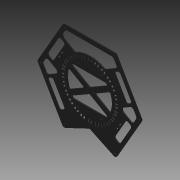
# Autodesk Inventor part: Bottom Plate
Saved by Autodesk Inventor 2015 (Build 190159000, 159)
## iProperties
Created: 2016-10-01
Part Number: Bottom Plate
Material: PVC, Unplasticized
Document SubType Name: Modeling
Designer: James Yelland
Density: 1.29 g/cm^3
Appearance: Smooth - White
Mass: 43.6601 g
Surface Area: 401.333 cm^2
Volume: 33.8451 cm^3
Author: James Yelland
Autodesk Inventor part; units mm, degrees
ref_plane "YZ Plane" through (0, 0, 0) normal (1, 0, 0) x (0, 1, 0)
ref_plane "XZ Plane" through (0, 0, 0) normal (0, 1, 0) x (-1, 0, 0)
ref_plane "XY Plane" through (0, 0, 0) normal (0, 0, 1) x (1, 0, 0)
sketch "Sketch1" plane through (0, 0, 0) normal (0, 1, 0) x (-1, 0, 0)
  line L0 (72.6878, -41.9663) -> (62.1878, -60.1529)
  line L1 (72.6878, -41.9663) -> (83.1878, -23.7798)
  line L2 (81.7237, -18.3157) -> (77.3936, -15.8157)
  line L3 (71.9295, -17.2797) -> (50.9295, -53.6529)
  line L4 (52.3936, -59.117) -> (56.7237, -61.617)
  arc A0 (56.7237, -61.617) -> (62.1878, -60.1529) centre (58.7237, -58.1529) ccw
  arc A1 (50.9295, -53.6529) -> (52.3936, -59.117) centre (54.3936, -55.6529) ccw
  arc A2 (77.3936, -15.8157) -> (71.9295, -17.2797) centre (75.3936, -19.2798) ccw
  arc A3 (83.1878, -23.7798) -> (81.7237, -18.3157) centre (79.7237, -21.7798) ccw
  line L5 (55.5994, -35.5644) -> (57.3314, -36.5644)
  line L6 (57.3314, -36.5644) -> (54.8314, -40.8945)
  line L7 (53.0994, -39.8945) -> (55.5994, -35.5644)
  line L8 (54.8314, -40.8945) -> (53.0994, -39.8945)
  line L9 (61.0994, -26.0381) -> (58.5994, -30.3683)
  line L10 (60.3314, -31.3683) -> (62.8314, -27.0381)
  line L11 (58.5994, -30.3683) -> (60.3314, -31.3683)
  line L12 (62.8314, -27.0381) -> (61.0994, -26.0381)
  line L13 (-72.6878, -41.9663) -> (-83.1878, -23.7798)
  line L14 (-72.6878, -41.9663) -> (-62.1878, -60.1529)
  line L15 (-56.7237, -61.617) -> (-52.3936, -59.117)
  line L16 (-50.9295, -53.6529) -> (-71.9294, -17.28)
  line L17 (-77.3936, -15.8157) -> (-81.7237, -18.3157)
  arc A4 (-81.7237, -18.3157) -> (-83.1878, -23.7798) centre (-79.7237, -21.7798) ccw
  arc A5 (-71.9294, -17.28) -> (-77.3936, -15.8157) centre (-75.3936, -19.2798) ccw
  arc A6 (-52.3936, -59.117) -> (-50.9295, -53.6529) centre (-54.3936, -55.6529) ccw
  arc A7 (-62.1878, -60.1529) -> (-56.7237, -61.617) centre (-58.7237, -58.1529) ccw
  line L18 (-58.5994, -30.3683) -> (-60.3314, -31.3683)
  line L19 (-61.0994, -26.0381) -> (-58.5994, -30.3683)
  line L20 (-62.8314, -27.0381) -> (-61.0994, -26.0381)
  line L21 (-60.3314, -31.3683) -> (-62.8314, -27.0381)
  line L22 (-54.8314, -40.8945) -> (-53.0994, -39.8945)
  line L23 (-53.0994, -39.8945) -> (-55.5994, -35.5644)
  line L24 (-55.5994, -35.5644) -> (-57.3314, -36.5644)
  line L25 (-57.3314, -36.5644) -> (-54.8314, -40.8945)
  line L26 (103.5566, -2.5) -> (54.8095, -86.9325)
  line L27 (-54.8095, -86.9325) -> (-103.5566, -2.5)
  line L28 (-103.5566, 2.5) -> (-53.9434, 88.4327)
  line L29 (-49.6132, 90.9327) -> (49.6132, 90.9327)
  line L30 (53.9434, 88.4327) -> (103.5566, 2.5)
  line L31 (2.1497, -66.9563) -> (48.3297, -88.9468)
  line L32 (-2.1497, -66.9563) -> (-48.3297, -88.9468)
  arc A8 (48.3297, -88.9468) -> (54.8095, -86.9325) centre (50.4794, -84.4325) ccw
  arc A9 (2.1497, -66.9563) -> (-2.1497, -66.9563) centre (0, -71.4706) ccw
  arc A10 (-54.8095, -86.9325) -> (-48.3297, -88.9468) centre (-50.4794, -84.4325) ccw
  arc A11 (-103.5566, 2.5) -> (-103.5566, -2.5) centre (-99.2265, 0) ccw
  arc A12 (-49.6132, 90.9327) -> (-53.9434, 88.4327) centre (-49.6132, 85.9327) ccw
  arc A13 (53.9434, 88.4327) -> (49.6132, 90.9327) centre (49.6132, 85.9327) ccw
  arc A14 (103.5566, -2.5) -> (103.5566, 2.5) centre (99.2265, 0) ccw
  circle A15 centre (49.6132, 85.9327) radius 1.6
  circle A16 centre (-49.6132, 85.9327) radius 1.6
  circle A17 centre (-99.2265, 0) radius 1.6
  circle A18 centre (99.2265, 0) radius 1.6
  arc A19 (48.9434, 79.7724) -> (44.6132, 82.2724) centre (44.6132, 77.2724) ccw
  arc A20 (-88.75, -10.8253) -> (-81.9199, -12.6554) centre (-84.4199, -8.3253) ccw
  arc A21 (-93.5566, 2.5) -> (-93.5566, -2.5) centre (-89.2265, 0) ccw
  arc A22 (81.9199, -12.6554) -> (88.75, -10.8253) centre (84.4199, -8.3253) ccw
  arc A23 (-44.6132, 82.2724) -> (-48.9434, 79.7724) centre (-44.6132, 77.2724) ccw
  arc A24 (93.5566, -2.5) -> (93.5566, 2.5) centre (89.2265, 0) ccw
  circle A25 centre (50.4794, -84.4325) radius 1.6
  circle A26 centre (-50.4794, -84.4325) radius 1.6
  line L33 (1.5, -53.75) -> (1.5, -56.75)
  line L34 (1.5, -56.75) -> (4.5, -56.75)
  line L35 (4.5, -56.75) -> (4.5, -50.75)
  line L36 (4.5, -50.75) -> (1.5, -50.75)
  line L37 (1.5, -50.75) -> (1.5, -53.75)
  line L38 (-1.5, -53.75) -> (-1.5, -56.75)
  line L39 (-1.5, -56.75) -> (-4.5, -56.75)
  line L40 (-1.5, -53.75) -> (-1.5, -53.75)
  line L41 (-1.5, -53.75) -> (-1.5, -50.75)
  line L42 (-1.5, -50.75) -> (-4.5, -50.75)
  line L43 (-4.5, -56.75) -> (-4.5, -50.75)
  line L44 (15.3604, -51.5303) -> (16.1369, -54.4281)
  line L45 (16.1369, -54.4281) -> (19.0346, -53.6516)
  line L46 (19.0346, -53.6516) -> (17.4817, -47.856)
  line L47 (17.4817, -47.856) -> (14.584, -48.6325)
  line L48 (14.584, -48.6325) -> (15.3604, -51.5303)
  line L49 (12.4626, -52.3067) -> (13.2391, -55.2045)
  line L50 (13.2391, -55.2045) -> (10.3413, -55.981)
  line L51 (12.4626, -52.3067) -> (11.6862, -49.409)
  line L52 (11.6862, -49.409) -> (8.7884, -50.1854)
  line L53 (10.3413, -55.981) -> (8.7884, -50.1854)
  line L54 (28.174, -45.7989) -> (29.674, -48.3969)
  line L55 (29.674, -48.3969) -> (32.2721, -46.8969)
  line L56 (32.2721, -46.8969) -> (29.2721, -41.7008)
  line L57 (29.2721, -41.7008) -> (26.674, -43.2008)
  line L58 (26.674, -43.2008) -> (28.174, -45.7989)
  line L59 (25.576, -47.2989) -> (27.076, -49.8969)
  line L60 (27.076, -49.8969) -> (24.4779, -51.3969)
  line L61 (25.576, -47.2989) -> (24.076, -44.7008)
  line L62 (24.076, -44.7008) -> (21.4779, -46.2008)
  line L63 (24.4779, -51.3969) -> (21.4779, -46.2008)
  line L64 (39.0676, -36.9463) -> (41.189, -39.0676)
  line L65 (41.189, -39.0676) -> (43.3103, -36.9463)
  line L66 (43.3103, -36.9463) -> (39.0676, -32.7037)
  line L67 (39.0676, -32.7037) -> (36.9463, -34.825)
  line L68 (36.9463, -34.825) -> (39.0676, -36.9463)
  line L69 (36.9463, -39.0676) -> (39.0676, -41.189)
  line L70 (39.0676, -41.189) -> (36.9463, -43.3103)
  line L71 (36.9463, -39.0676) -> (34.825, -36.9463)
  line L72 (34.825, -36.9463) -> (32.7037, -39.0676)
  line L73 (36.9463, -43.3103) -> (32.7037, -39.0676)
  line L74 (47.2989, -25.576) -> (49.8969, -27.076)
  line L75 (49.8969, -27.076) -> (51.3969, -24.4779)
  line L76 (51.3969, -24.4779) -> (46.2008, -21.4779)
  line L77 (46.2008, -21.4779) -> (44.7008, -24.076)
  line L78 (44.7008, -24.076) -> (47.2989, -25.576)
  line L79 (45.7989, -28.174) -> (48.3969, -29.674)
  line L80 (48.3969, -29.674) -> (46.8969, -32.2721)
  line L81 (45.7989, -28.174) -> (43.2008, -26.674)
  line L82 (43.2008, -26.674) -> (41.7008, -29.2721)
  line L83 (46.8969, -32.2721) -> (41.7008, -29.2721)
  line L84 (52.3067, -12.4626) -> (55.2045, -13.2391)
  line L85 (55.2045, -13.2391) -> (55.981, -10.3413)
  line L86 (55.981, -10.3413) -> (50.1854, -8.7884)
  line L87 (50.1854, -8.7884) -> (49.409, -11.6862)
  line L88 (49.409, -11.6862) -> (52.3067, -12.4626)
  line L89 (51.5303, -15.3604) -> (54.4281, -16.1369)
  line L90 (54.4281, -16.1369) -> (53.6516, -19.0346)
  line L91 (51.5303, -15.3604) -> (48.6325, -14.584)
  line L92 (48.6325, -14.584) -> (47.856, -17.4817)
  line L93 (53.6516, -19.0346) -> (47.856, -17.4817)
  line L94 (53.75, 1.5) -> (56.75, 1.5)
  line L95 (56.75, 1.5) -> (56.75, 4.5)
  line L96 (56.75, 4.5) -> (50.75, 4.5)
  line L97 (50.75, 4.5) -> (50.75, 1.5)
  line L98 (50.75, 1.5) -> (53.75, 1.5)
  line L99 (53.75, -1.5) -> (56.75, -1.5)
  line L100 (56.75, -1.5) -> (56.75, -4.5)
  line L101 (53.75, -1.5) -> (50.75, -1.5)
  line L102 (50.75, -1.5) -> (50.75, -4.5)
  line L103 (56.75, -4.5) -> (50.75, -4.5)
  line L104 (51.5303, 15.3604) -> (54.4281, 16.1369)
  line L105 (54.4281, 16.1369) -> (53.6516, 19.0346)
  line L106 (53.6516, 19.0346) -> (47.856, 17.4817)
  line L107 (47.856, 17.4817) -> (48.6325, 14.584)
  line L108 (48.6325, 14.584) -> (51.5303, 15.3604)
  line L109 (52.3067, 12.4626) -> (55.2045, 13.2391)
  line L110 (55.2045, 13.2391) -> (55.981, 10.3413)
  line L111 (52.3067, 12.4626) -> (49.409, 11.6862)
  line L112 (49.409, 11.6862) -> (50.1854, 8.7884)
  line L113 (55.981, 10.3413) -> (50.1854, 8.7884)
  line L114 (45.7989, 28.174) -> (48.3969, 29.674)
  line L115 (48.3969, 29.674) -> (46.8969, 32.2721)
  line L116 (46.8969, 32.2721) -> (41.7008, 29.2721)
  line L117 (41.7008, 29.2721) -> (43.2008, 26.674)
  line L118 (43.2008, 26.674) -> (45.7989, 28.174)
  line L119 (47.2989, 25.576) -> (49.8969, 27.076)
  line L120 (49.8969, 27.076) -> (51.3969, 24.4779)
  line L121 (47.2989, 25.576) -> (44.7008, 24.076)
  line L122 (44.7008, 24.076) -> (46.2008, 21.4779)
  line L123 (51.3969, 24.4779) -> (46.2008, 21.4779)
  line L124 (36.9463, 39.0676) -> (39.0676, 41.189)
  line L125 (39.0676, 41.189) -> (36.9463, 43.3103)
  line L126 (36.9463, 43.3103) -> (32.7037, 39.0676)
  line L127 (32.7037, 39.0676) -> (34.825, 36.9463)
  line L128 (34.825, 36.9463) -> (36.9463, 39.0676)
  line L129 (39.0676, 36.9463) -> (41.189, 39.0676)
  line L130 (41.189, 39.0676) -> (43.3103, 36.9463)
  line L131 (39.0676, 36.9463) -> (36.9463, 34.825)
  line L132 (36.9463, 34.825) -> (39.0676, 32.7037)
  line L133 (43.3103, 36.9463) -> (39.0676, 32.7037)
  line L134 (25.576, 47.2989) -> (27.076, 49.8969)
  line L135 (27.076, 49.8969) -> (24.4779, 51.3969)
  line L136 (24.4779, 51.3969) -> (21.4779, 46.2008)
  line L137 (21.4779, 46.2008) -> (24.076, 44.7008)
  line L138 (24.076, 44.7008) -> (25.576, 47.2989)
  line L139 (28.174, 45.7989) -> (29.674, 48.3969)
  line L140 (29.674, 48.3969) -> (32.2721, 46.8969)
  line L141 (28.174, 45.7989) -> (26.674, 43.2008)
  line L142 (26.674, 43.2008) -> (29.2721, 41.7008)
  line L143 (32.2721, 46.8969) -> (29.2721, 41.7008)
  line L144 (12.4626, 52.3067) -> (13.2391, 55.2045)
  line L145 (13.2391, 55.2045) -> (10.3413, 55.981)
  line L146 (10.3413, 55.981) -> (8.7884, 50.1854)
  line L147 (8.7884, 50.1854) -> (11.6862, 49.409)
  line L148 (11.6862, 49.409) -> (12.4626, 52.3067)
  line L149 (15.3604, 51.5303) -> (16.1369, 54.4281)
  line L150 (16.1369, 54.4281) -> (19.0346, 53.6516)
  line L151 (15.3604, 51.5303) -> (14.584, 48.6325)
  line L152 (14.584, 48.6325) -> (17.4817, 47.856)
  line L153 (19.0346, 53.6516) -> (17.4817, 47.856)
  line L154 (-1.5, 53.75) -> (-1.5, 56.75)
  line L155 (-1.5, 56.75) -> (-4.5, 56.75)
  line L156 (-4.5, 56.75) -> (-4.5, 50.75)
  line L157 (-4.5, 50.75) -> (-1.5, 50.75)
  line L158 (-1.5, 50.75) -> (-1.5, 53.75)
  line L159 (1.5, 53.75) -> (1.5, 56.75)
  line L160 (1.5, 56.75) -> (4.5, 56.75)
  line L161 (1.5, 53.75) -> (1.5, 50.75)
  line L162 (1.5, 50.75) -> (4.5, 50.75)
  line L163 (4.5, 56.75) -> (4.5, 50.75)
  line L164 (-15.3604, 51.5303) -> (-16.1369, 54.4281)
  line L165 (-16.1369, 54.4281) -> (-19.0346, 53.6516)
  line L166 (-19.0346, 53.6516) -> (-17.4817, 47.856)
  line L167 (-17.4817, 47.856) -> (-14.584, 48.6325)
  line L168 (-14.584, 48.6325) -> (-15.3604, 51.5303)
  line L169 (-12.4626, 52.3067) -> (-13.2391, 55.2045)
  line L170 (-13.2391, 55.2045) -> (-10.3413, 55.981)
  line L171 (-12.4626, 52.3067) -> (-11.6862, 49.409)
  line L172 (-11.6862, 49.409) -> (-8.7884, 50.1854)
  line L173 (-10.3413, 55.981) -> (-8.7884, 50.1854)
  line L174 (-28.174, 45.7989) -> (-29.674, 48.3969)
  line L175 (-29.674, 48.3969) -> (-32.2721, 46.8969)
  line L176 (-32.2721, 46.8969) -> (-29.2721, 41.7008)
  line L177 (-29.2721, 41.7008) -> (-26.674, 43.2008)
  line L178 (-26.674, 43.2008) -> (-28.174, 45.7989)
  line L179 (-25.576, 47.2989) -> (-27.076, 49.8969)
  line L180 (-27.076, 49.8969) -> (-24.4779, 51.3969)
  line L181 (-25.576, 47.2989) -> (-24.076, 44.7008)
  line L182 (-24.076, 44.7008) -> (-21.4779, 46.2008)
  line L183 (-24.4779, 51.3969) -> (-21.4779, 46.2008)
  line L184 (-39.0676, 36.9463) -> (-41.189, 39.0676)
  line L185 (-41.189, 39.0676) -> (-43.3103, 36.9463)
  line L186 (-43.3103, 36.9463) -> (-39.0676, 32.7037)
  line L187 (-39.0676, 32.7037) -> (-36.9463, 34.825)
  line L188 (-36.9463, 34.825) -> (-39.0676, 36.9463)
  line L189 (-36.9463, 39.0676) -> (-39.0676, 41.189)
  line L190 (-39.0676, 41.189) -> (-36.9463, 43.3103)
  line L191 (-36.9463, 39.0676) -> (-34.825, 36.9463)
  line L192 (-34.825, 36.9463) -> (-32.7037, 39.0676)
  line L193 (-36.9463, 43.3103) -> (-32.7037, 39.0676)
  line L194 (-47.2989, 25.576) -> (-49.8969, 27.076)
  line L195 (-49.8969, 27.076) -> (-51.3969, 24.4779)
  line L196 (-51.3969, 24.4779) -> (-46.2008, 21.4779)
  line L197 (-46.2008, 21.4779) -> (-44.7008, 24.076)
  line L198 (-44.7008, 24.076) -> (-47.2989, 25.576)
  line L199 (-45.7989, 28.174) -> (-48.3969, 29.674)
  line L200 (-48.3969, 29.674) -> (-46.8969, 32.2721)
  line L201 (-45.7989, 28.174) -> (-43.2008, 26.674)
  line L202 (-43.2008, 26.674) -> (-41.7008, 29.2721)
  line L203 (-46.8969, 32.2721) -> (-41.7008, 29.2721)
  line L204 (-52.3067, 12.4626) -> (-55.2045, 13.2391)
  line L205 (-55.2045, 13.2391) -> (-55.981, 10.3413)
  line L206 (-55.981, 10.3413) -> (-50.1854, 8.7884)
  line L207 (-50.1854, 8.7884) -> (-49.409, 11.6862)
  line L208 (-49.409, 11.6862) -> (-52.3067, 12.4626)
  line L209 (-51.5303, 15.3604) -> (-54.4281, 16.1369)
  line L210 (-54.4281, 16.1369) -> (-53.6516, 19.0346)
  line L211 (-51.5303, 15.3604) -> (-48.6325, 14.584)
  line L212 (-48.6325, 14.584) -> (-47.856, 17.4817)
  line L213 (-53.6516, 19.0346) -> (-47.856, 17.4817)
  line L214 (-53.75, -1.5) -> (-56.75, -1.5)
  line L215 (-56.75, -1.5) -> (-56.75, -4.5)
  line L216 (-56.75, -4.5) -> (-50.75, -4.5)
  line L217 (-50.75, -4.5) -> (-50.75, -1.5)
  line L218 (-50.75, -1.5) -> (-53.75, -1.5)
  line L219 (-53.75, 1.5) -> (-56.75, 1.5)
  line L220 (-56.75, 1.5) -> (-56.75, 4.5)
  line L221 (-53.75, 1.5) -> (-50.75, 1.5)
  line L222 (-50.75, 1.5) -> (-50.75, 4.5)
  line L223 (-56.75, 4.5) -> (-50.75, 4.5)
  line L224 (-51.5303, -15.3604) -> (-54.4281, -16.1369)
  line L225 (-54.4281, -16.1369) -> (-53.6516, -19.0346)
  line L226 (-53.6516, -19.0346) -> (-47.856, -17.4817)
  line L227 (-47.856, -17.4817) -> (-48.6325, -14.584)
  line L228 (-48.6325, -14.584) -> (-51.5303, -15.3604)
  line L229 (-52.3067, -12.4626) -> (-55.2045, -13.2391)
  line L230 (-55.2045, -13.2391) -> (-55.981, -10.3413)
  line L231 (-52.3067, -12.4626) -> (-49.409, -11.6862)
  line L232 (-49.409, -11.6862) -> (-50.1854, -8.7884)
  line L233 (-55.981, -10.3413) -> (-50.1854, -8.7884)
  line L234 (-45.7989, -28.174) -> (-48.3969, -29.674)
  line L235 (-48.3969, -29.674) -> (-46.8969, -32.2721)
  line L236 (-46.8969, -32.2721) -> (-41.7008, -29.2721)
  line L237 (-41.7008, -29.2721) -> (-43.2008, -26.674)
  line L238 (-43.2008, -26.674) -> (-45.7989, -28.174)
  line L239 (-47.2989, -25.576) -> (-49.8969, -27.076)
  line L240 (-49.8969, -27.076) -> (-51.3969, -24.4779)
  line L241 (-47.2989, -25.576) -> (-44.7008, -24.076)
  line L242 (-44.7008, -24.076) -> (-46.2008, -21.4779)
  line L243 (-51.3969, -24.4779) -> (-46.2008, -21.4779)
  line L244 (-36.9463, -39.0676) -> (-39.0676, -41.189)
  line L245 (-39.0676, -41.189) -> (-36.9463, -43.3103)
  line L246 (-36.9463, -43.3103) -> (-32.7037, -39.0676)
  line L247 (-32.7037, -39.0676) -> (-34.825, -36.9463)
  line L248 (-34.825, -36.9463) -> (-36.9463, -39.0676)
  line L249 (-39.0676, -36.9463) -> (-41.189, -39.0676)
  line L250 (-41.189, -39.0676) -> (-43.3103, -36.9463)
  line L251 (-39.0676, -36.9463) -> (-36.9463, -34.825)
  line L252 (-36.9463, -34.825) -> (-39.0676, -32.7037)
  line L253 (-43.3103, -36.9463) -> (-39.0676, -32.7037)
  line L254 (-25.576, -47.2989) -> (-27.076, -49.8969)
  line L255 (-27.076, -49.8969) -> (-24.4779, -51.3969)
  line L256 (-24.4779, -51.3969) -> (-21.4779, -46.2008)
  line L257 (-21.4779, -46.2008) -> (-24.076, -44.7008)
  line L258 (-24.076, -44.7008) -> (-25.576, -47.2989)
  line L259 (-28.174, -45.7989) -> (-29.674, -48.3969)
  line L260 (-29.674, -48.3969) -> (-32.2721, -46.8969)
  line L261 (-28.174, -45.7989) -> (-26.674, -43.2008)
  line L262 (-26.674, -43.2008) -> (-29.2721, -41.7008)
  line L263 (-32.2721, -46.8969) -> (-29.2721, -41.7008)
  line L264 (-12.4626, -52.3067) -> (-13.2391, -55.2045)
  line L265 (-13.2391, -55.2045) -> (-10.3413, -55.981)
  line L266 (-10.3413, -55.981) -> (-8.7884, -50.1854)
  line L267 (-8.7884, -50.1854) -> (-11.6862, -49.409)
  line L268 (-11.6862, -49.409) -> (-12.4626, -52.3067)
  line L269 (-15.3604, -51.5303) -> (-16.1369, -54.4281)
  line L270 (-16.1369, -54.4281) -> (-19.0346, -53.6516)
  line L271 (-15.3604, -51.5303) -> (-14.584, -48.6325)
  line L272 (-14.584, -48.6325) -> (-17.4817, -47.856)
  line L273 (-19.0346, -53.6516) -> (-17.4817, -47.856)
  arc A27 (-83.1878, 23.7798) -> (-81.7237, 18.3157) centre (-79.7237, 21.7798) ccw
  line L274 (-81.7237, 18.3157) -> (-77.3936, 15.8157)
  arc A28 (-77.3936, 15.8157) -> (-71.9295, 17.2798) centre (-75.3936, 19.2798) ccw
  line L275 (-72.6878, 41.9663) -> (-83.1878, 23.7798)
  line L276 (-62.8314, 27.0381) -> (-61.0994, 26.0381)
  line L277 (-60.3314, 31.3683) -> (-62.8314, 27.0381)
  line L278 (-61.0994, 26.0381) -> (-58.5994, 30.3683)
  line L279 (-58.5994, 30.3683) -> (-60.3314, 31.3683)
  line L280 (-55.5994, 35.5644) -> (-57.3314, 36.5644)
  line L281 (-57.3314, 36.5644) -> (-54.8314, 40.8945)
  line L282 (-53.0994, 39.8945) -> (-55.5994, 35.5644)
  line L283 (-71.9295, 17.2798) -> (-50.9296, 53.6527)
  line L284 (-72.6878, 41.9663) -> (-62.1878, 60.1529)
  line L285 (-54.8314, 40.8945) -> (-53.0994, 39.8945)
  arc A29 (-56.7237, 61.617) -> (-62.1878, 60.1529) centre (-58.7237, 58.1529) ccw
  line L286 (-52.3936, 59.117) -> (-56.7237, 61.617)
  arc A30 (-50.9296, 53.6527) -> (-52.3936, 59.117) centre (-54.3936, 55.6529) ccw
  arc A31 (-53.75, 71.4471) -> (-51.9199, 64.617) centre (-49.4199, 68.9471) ccw
  arc A32 (-81.9199, 12.6554) -> (-88.75, 10.8253) centre (-84.4199, 8.3253) ccw
  arc A33 (-31.4758, 52.8136) -> (-28.5484, 52.773) centre (-29.9758, 55.4117) ccw
  arc A34 (62.1878, 60.1529) -> (56.7237, 61.6169) centre (58.7237, 58.1528) ccw
  line L287 (56.7237, 61.6169) -> (52.3936, 59.1169)
  arc A35 (52.3936, 59.1169) -> (50.9295, 53.6528) centre (54.3936, 55.6528) ccw
  line L288 (72.6878, 41.9663) -> (62.1878, 60.1529)
  line L289 (54.8314, 40.8945) -> (53.0994, 39.8945)
  line L290 (57.3314, 36.5644) -> (54.8314, 40.8945)
  line L291 (53.0994, 39.8945) -> (55.5994, 35.5644)
  line L292 (55.5994, 35.5644) -> (57.3314, 36.5644)
  line L293 (58.5994, 30.3683) -> (60.3314, 31.3683)
  line L294 (60.3314, 31.3683) -> (62.8314, 27.0381)
  line L295 (61.0994, 26.0381) -> (58.5994, 30.3683)
  line L296 (50.9295, 53.6528) -> (71.9295, 17.2798)
  line L297 (72.6878, 41.9663) -> (83.1878, 23.7798)
  line L298 (62.8314, 27.0381) -> (61.0994, 26.0381)
  arc A36 (81.7237, 18.3157) -> (83.1878, 23.7798) centre (79.7237, 21.7798) ccw
  line L299 (77.3936, 15.8157) -> (81.7237, 18.3157)
  arc A37 (71.9295, 17.2798) -> (77.3936, 15.8157) centre (75.3936, 19.2798) ccw
  arc A38 (88.75, 10.8253) -> (81.9199, 12.6554) centre (84.4199, 8.3253) ccw
  arc A39 (51.9199, 64.617) -> (53.75, 71.4471) centre (49.4199, 68.9471) ccw
  line L300 (51.9199, 64.617) -> (31.4758, 52.8136)
  arc A40 (28.5484, 52.773) -> (31.4758, 52.8136) centre (29.9758, 55.4117) ccw
  arc A41 (67.5, 4.3301) -> (67.5, -4.3301) centre (70, 0) ccw
  arc A42 (-67.5, -4.3301) -> (-67.5, 4.3301) centre (-70, 0) ccw
  line L301 (53.75, 71.4471) -> (48.9434, 79.7724)
  line L302 (44.6132, 82.2724) -> (-44.6132, 82.2724)
  line L303 (-48.9434, 79.7724) -> (-53.75, 71.4471)
  line L304 (-51.9199, 64.617) -> (-31.4758, 52.8136)
  arc A43 (28.5484, 52.773) -> (-28.5484, 52.773) centre (0, 0) ccw
  line L305 (-67.5, -4.3301) -> (-81.9199, -12.6554)
  line L306 (-88.75, -10.8253) -> (-93.5566, -2.5)
  line L307 (-93.5566, 2.5) -> (-88.75, 10.8253)
  line L308 (-81.9199, 12.6554) -> (-67.5, 4.3301)
  line L309 (81.9199, 12.6554) -> (67.5, 4.3301)
  line L310 (67.5, -4.3301) -> (81.9199, -12.6554)
  line L311 (88.75, -10.8253) -> (93.5566, -2.5)
  line L312 (93.5566, 2.5) -> (88.75, 10.8253)
  line L313 (0, 30) -> (-31.225, 30)
  line L314 (0, 30) -> (31.225, 30)
  line L315 (0, -30) -> (-31.225, -30)
  line L316 (0, -30) -> (31.225, -30)
  arc A44 (42.1141, -15.8557) -> (42.1141, 15.8557) centre (0, 0) ccw
  arc A45 (-42.1141, 15.8558) -> (-42.1141, -15.8558) centre (0, 0) ccw
  arc A46 (34.525, 28.7563) -> (31.225, 30) centre (31.225, 25) ccw
  arc A47 (-31.225, 30) -> (-34.525, 28.7563) centre (-31.225, 25) ccw
  arc A48 (-34.525, -28.7563) -> (-31.225, -30) centre (-31.225, -25) ccw
  arc A49 (31.225, -30) -> (34.525, -28.7563) centre (31.225, -25) ccw
  circle A50 centre (22.6343, 38) radius 1.6
  circle A51 centre (-22.6343, 38) radius 1.6
  circle A52 centre (-22.6343, -38) radius 1.6
  circle A53 centre (22.6343, -38) radius 1.6
  line L317 (61.4295, 35.4663) -> (63.9295, 31.1362)
  line L318 (39.2424, -16.8831) -> (13, -1.7321)
  line L319 (39.2424, 16.8831) -> (13, 1.7321)
  line L320 (34.205, 25.5218) -> (1, 6.3509)
  line L321 (-1, 6.3509) -> (-34.205, 25.5218)
  line L322 (-39.2423, 16.8832) -> (-12.9998, 1.7321)
  line L323 (-12.9998, -1.7321) -> (-39.2423, -16.8832)
  line L324 (-34.205, -25.5218) -> (-1, -6.3509)
  line L325 (1, -6.3509) -> (34.205, -25.5218)
  arc A54 (-1, 6.3509) -> (1, 6.3509) centre (0, 8.0829) ccw
  arc A55 (-12.9998, -1.7321) -> (-12.9998, 1.7321) centre (-13.9998, 0) ccw
  arc A56 (1, -6.3509) -> (-1, -6.3509) centre (0, -8.0829) ccw
  arc A57 (13, 1.7321) -> (13, -1.7321) centre (14, 0) ccw
  arc A58 (39.2424, -16.8831) -> (42.1141, -15.8557) centre (40.2424, -15.151) ccw
  arc A59 (34.525, -28.7563) -> (34.205, -25.5218) centre (33.205, -27.2538) ccw
  arc A60 (-42.1141, -15.8558) -> (-39.2423, -16.8832) centre (-40.2423, -15.1511) ccw
  arc A61 (-34.205, -25.5218) -> (-34.525, -28.7563) centre (-33.205, -27.2538) ccw
  arc A62 (-39.2423, 16.8832) -> (-42.1141, 15.8558) centre (-40.2423, 15.1511) ccw
  arc A63 (-34.525, 28.7563) -> (-34.205, 25.5218) centre (-33.205, 27.2538) ccw
  arc A64 (42.1141, 15.8557) -> (39.2424, 16.8831) centre (40.2424, 15.151) ccw
  arc A65 (34.205, 25.5218) -> (34.525, 28.7563) centre (33.205, 27.2538) ccw
  circle A66 centre (7, 0) radius 1.6
  circle A67 centre (-7, 0) radius 1.6
  point P0 (60.1878, -63.617)
  point P1 (85.1878, -20.3157)
  point P2 (73.9295, -13.8157)
  point P3 (48.9295, -57.117)
  point P4 (-85.1878, -20.3157)
  point P5 (-60.1878, -63.617)
  point P6 (-48.9295, -57.117)
  point P7 (-73.9295, -13.8157)
  point P8 (105, 0)
  point P9 (52.5, -90.9327)
  point P10 (-105, 0)
  point P11 (-52.5, 90.9327)
  point P12 (52.5, 90.9327)
  point P13 (-86.25, -15.1554)
  point P14 (60, 0)
  point P15 (-60, 0)
  point P16 (-73.9295, 13.8157)
  point P17 (-85.1878, 20.3157)
  point P18 (-48.9295, 57.117)
  point P19 (-60.1878, 63.617)
  point P20 (-30, 51.9615)
  point P21 (-60, 0)
  point P22 (48.9295, 57.1169)
  point P23 (60.1878, 63.6169)
  point P24 (73.9295, 13.8157)
  point P25 (85.1878, 20.3157)
  point P26 (60, 0)
  point P27 (30, 51.9615)
  point P28 (-33.541, 30)
  point P29 (33.541, 30)
  point P30 (-33.541, -30)
  point P31 (33.541, -30)
  point P32 (41.2298, -18.0305)
  point P33 (41.2298, 18.0305)
  point P34 (-41.2298, 18.0306)
  point P35 (-41.2298, -18.0306)
  dimension "d11" = 360
  dimension "d30" = 360
  dimension "d32" = 5
  dimension "d82" = 5
  dimension "d86" = 5
  dimension "d87" = 3.2
  dimension "d91" = 5
  dimension "d94" = 2
  dimension "d95" = 2
  dimension "d98" = 3.2
  constraints: 652 end point, 120 point on circle, 77 point on line, 68 centre point, 33 tangent, 13 equal radius, 8 coincident, 6 perpendicular, 1 horizontal, 1 midpoint, 1 parallel
  measures "d32" radius of A23
  measures "d82" radius of A41
  measures "d86" radius of A46
  measures "d87" diameter of A50
  measures "d91" distance of L317.start L317.end
  measures "d94" radius of A60
  measures "d95" radius of A63
  measures "d98" diameter of A66
extrude "Extrusion1" add sketch "Sketch1" along normal blind 2
body "Solid1"
